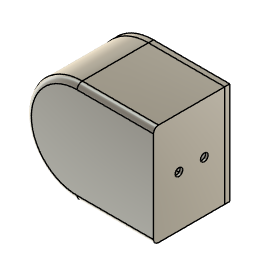
TRARM02_Link4 (Autodesk Fusion 360 design; units mm, degrees)
Autodesk Fusion 360 part; units mm, degrees
sketch "스케치1" plane through (0, 0, 0) normal (0, 0, 1) x (1, 0, 0) in component "TRARM02_Link4A_30x40x2 v1"
  line L0 (20, 30) -> (20, 0)
  line L1 (-20, 30) -> (-20, 0)
  arc A0 (-20, 0) -> (20, 0) centre (0, 0) ccw
  line L2 (-20, 30) -> (20, 30)
  dimension "d1" = 40
  dimension "d128" = 30
  dimension "d129" = 20
  constraint coincident A0.centre origin
  constraint tangent L0 A0
  constraint vertical L0
  constraint parallel L0 L1
  constraint horizontal L0.start L1.start
  measures "d1" diameter of A0
  measures "d128" vertical distance of A0.centre L1.start
  measures "d129" distance of A0.centre L1
extrude "돌출1" add sketch "스케치1" along normal blind 2 makes body 1 in component "TRARM02_Link4A_30x40x2 v1"
sketch "스케치2" plane through (0, 0, 2) normal (0, 0, 1) x (-1, 0, 0) in component "TRARM02_Link4A_30x40x2 v1"
  circle A0 centre (0, 8.75) radius 1.1
  circle A1 centre (0, -19.05) radius 1.1
  line L0 (6.1, -16.65) -> (-6.1, -16.65)
  line L1 (-6.1, -16.65) -> (-6.1, 6.35)
  line L2 (-6.1, 6.35) -> (6.1, 6.35)
  line L3 (6.1, 6.35) -> (6.1, -16.65)
  dimension "d7" = 2.2
  dimension "d8" = 27.8
  dimension "d9" = 8.75
  dimension "d11" = 23
  dimension "d12" = 2.4
  dimension "d13" = 12.2
  dimension "d14" = 6.1
  constraint equal A0 A1
  constraint horizontal L0
  constraint vertical L1
  constraint horizontal L2
  constraint vertical L3
  constraint vertical origin A0.centre
  constraint vertical origin A1.centre
  measures "d7" diameter of A0
  measures "d8" distance of A0.centre A1.centre
  measures "d9" distance of origin A0.centre
  measures "d11" distance of L0.end L1.end
  measures "d12" vertical distance of A1.centre L0.end
  measures "d13" distance of L0.start L0.end
  measures "d14" horizontal distance of origin L1.end
extrude "돌출2" cut sketch "스케치2" against normal blind 2 bodies 1 in component "TRARM02_Link4A_30x40x2 v1"
chamfer "챔퍼2" distance 1.5 angle 45 2 edges at (1.0256, 19.4478, 0) (1.0256, -8.3522, 0) on bodies 1 in component "TRARM02_Link4A_30x40x2 v1"
sketch "스케치14" plane through (0, 0, 2) normal (0, 0, 1) x (-1, 0, 0) in component "TRARM02_Link4A_30x40x2 v1"
  line L0 (20, -30) -> (20, 0) construction
  line L1 (-20, 0) -> (-20, -30) construction
  arc A0 (20, 0) -> (-20, 0) centre (0, 0) ccw construction
  line L2 (19, -29) -> (19, 0)
  arc A1 (19, 0) -> (-19, 0) centre (0, 0) ccw
  line L3 (-19, 0) -> (-19, -29)
  line L4 (-15, -6) -> (-18, -6)
  line L5 (15, -6) -> (18, -6)
  line L6 (15, 0) -> (18, 0)
  arc A2 (15, 0) -> (15, -6) centre (15, -3) ccw
  line L7 (18, -28) -> (18, -6)
  line L8 (-18, -6) -> (-18, -28)
  line L9 (-15, 0) -> (-18, 0)
  arc A3 (18, 0) -> (-18, 0) centre (0, 0) ccw
  arc A4 (-15, -6) -> (-15, 0) centre (-15, -3) ccw
  line L10 (-20, -30) -> (20, -30)
  line L11 (18, -28) -> (-18, -28)
  line L12 (19, -29) -> (-19, -29)
  dimension "d112" = 3
  dimension "d113" = 3
  dimension "d120" = 3
  dimension "d121" = 1
  dimension "d124" = 6
  dimension "d125" = 6
  dimension "d126" = 3
  dimension "d130" = 1
  dimension "d131" = 1
  constraint coincident L6.end L7
  constraint perpendicular L6 L7
  constraint coincident L6 A2.start
  constraint horizontal L5
  constraint vertical L6.start A2.centre
  constraint coincident L6.start A2.start
  constraint horizontal L4
  constraint horizontal L9
  constraint vertical L8
  constraint equal L4 L9
  constraint vertical L4.end L9.end
  constraint coincident A0.centre L6
  constraint coincident A0.centre L9
  constraint concentric A0 A3
  constraint concentric A0 A1
  constraint tangent L2 A1
  constraint tangent A1 L3
  constraint vertical L7
  constraint horizontal L12
  constraint horizontal L11
  measures "d112" distance of L5.start L5.end
  measures "d113" distance of L4.start L4.end
  measures "d120" distance of L6.start L6.end
  measures "d121" distance of L3 L8
  measures "d124" distance of A0.centre L5
  measures "d125" distance of A0.centre L4
  measures "d126" radius of A4
  measures "d130" distance of L11 L12
  measures "d131" distance of L10 L12
extrude "돌출15" add sketch "스케치14" along normal blind 2 bodies 1 in component "TRARM02_Link4A_30x40x2 v1"
sketch "스케치16" plane through (0, 0, 4) normal (0, 0, 1) x (-1, 0, 0) in component "TRARM02_Link4A_30x40x2 v1"
  circle A0 centre (-15, -3) radius 1.5
  circle A1 centre (15, -3) radius 1.5
  arc A2 (15, 0) -> (15, -6) centre (15, -3) ccw
  arc A3 (-15, -6) -> (-15, 0) centre (-15, -3) ccw
  dimension "d106" = 3
  constraint equal A0 A1
  constraint concentric A1 A2
  constraint concentric A0 A3
  measures "d106" diameter of A0
extrude "돌출17" cut sketch "스케치16" against normal blind 4 bodies 1 in component "TRARM02_Link4A_30x40x2 v1"
chamfer "챔퍼4" distance 2 angle 45 1 edges at (16.3985, 3.5424, 0) on bodies 1 in component "TRARM02_Link4A_30x40x2 v1"
chamfer "챔퍼4" distance 2 angle 45 1 edges at (-13.6015, 3.5424, 0) on bodies 1 in component "TRARM02_Link4A_30x40x2 v1"
move_body "이동1" bodies 1 to x (0, -1, 0) y (1, 0, 0) z (0, 0, 1) at (0, 0, 0) in component "TRARM02_Link4A_30x40x2 v1"
sketch "스케치1 (2)" plane through (0, 0, 0) normal (0, 0, 1) x (1, 0, 0) in component "TRARM02_Link4B_30x40x28 v1"
  line L0 (20, 30) -> (20, 0)
  line L1 (-20, 30) -> (-20, 0)
  arc A0 (-20, 0) -> (20, 0) centre (0, 0) ccw
  line L2 (-20, 30) -> (20, 30)
  dimension "d1_1" = 40
  dimension "d144" = 30
  constraint coincident A0.centre origin
  constraint tangent L0 A0
  constraint vertical L0
  constraint parallel L0 L1
  constraint horizontal L0.start L1.start
  measures "d1_1" diameter of A0
  measures "d144" vertical distance of A0.centre L1.start
extrude "돌출1'" add sketch "스케치1 (2)" along normal blind 2 separate body makes body 2 in component "TRARM02_Link4B_30x40x28 v1"
sketch "스케치14 (2)" plane through (0, 0, 2) normal (0, 0, 1) x (-1, 0, 0) in component "TRARM02_Link4B_30x40x28 v1"
  line L0 (20, -30) -> (20, 0)
  line L1 (-20, 0) -> (-20, -30)
  arc A0 (20, 0) -> (-20, 0) centre (0, 0) ccw
  arc A1 (19, 0) -> (-19, 0) centre (0, 0) ccw
  line L2 (15, -6) -> (19, -6)
  line L3 (15, 0) -> (19, 0)
  arc A2 (15, 0) -> (15, -6) centre (15, -3) ccw
  line L4 (-15, -6) -> (-19, -6)
  arc A3 (-15, -6) -> (-15, 0) centre (-15, -3) ccw
  line L5 (19, -29) -> (19, -6)
  line L6 (-19, -6) -> (-19, -29)
  line L7 (-15, 0) -> (-19, 0)
  line L8 (-20, -30) -> (20, -30)
  line L9 (20, -30) -> (-20, -30)
  line L10 (19, -29) -> (-19, -29)
  dimension "d111_1" = 15
  dimension "d112_1" = 6
  dimension "d114" = 3
  dimension "d132" = 4
  dimension "d133" = 4
  dimension "d134" = 4
  dimension "d135" = 1
  dimension "d136" = 4
  dimension "d142" = 1
  dimension "d143" = 19
  dimension "d145" = 1
  constraint concentric A0 A1
  constraint equal A2 A3
  constraint horizontal A2.centre A3.centre
  constraint horizontal L7
  constraint vertical L6
  constraint horizontal L4
  constraint vertical L5
  constraint horizontal L3
  constraint coincident A1.start L3.end
  constraint horizontal L2
  constraint coincident L0.start L8.end
  constraint coincident L1.end L8.start
  constraint horizontal L10
  measures "d111_1" horizontal distance of A0.centre A2.centre
  measures "d112_1" diameter of A2
  measures "d114" vertical distance of A0.centre A2.centre
  measures "d132" distance of L3.start A1.start
  measures "d133" distance of L2.start L2.end
  measures "d134" distance of A1.end A3.end
  measures "d135" distance of L1 L6
  measures "d136" distance of L4.start L4.end
  measures "d142" distance of L0 L5
  measures "d143" radius of A1
  measures "d145" distance of L9 L10
extrude "돌출18" add sketch "스케치14 (2)" along normal blind 26 bodies 2 in component "TRARM02_Link4B_30x40x28 v1"
sketch "스케치17" plane through (0, 0, 28) normal (0, 0, 1) x (-1, 0, 0) in component "TRARM02_Link4B_30x40x28 v1"
  line L0 (-19, -6) -> (-15, -6)
  line L1 (-15, 0) -> (-19, 0)
  arc A0 (-15, -6) -> (-15, 0) centre (-15, -3) ccw
  arc A1 (15, 0) -> (15, -6) centre (15, -3) ccw
  line L2 (19, 0) -> (15, 0)
  line L3 (15, -6) -> (19, -6)
  line L4 (19, -6) -> (19, 0)
  line L5 (-19, -6) -> (-19, 0)
  point P0 (15, 0)
  constraint coincident L3.end L4.start
  constraint coincident L2.start L4.end
  constraint coincident L0.start L5.start
  constraint coincident L1.end L5.end
extrude "돌출19" cut sketch "스케치17" against normal blind 2 bodies 2 in component "TRARM02_Link4B_30x40x28 v1"
sketch "스케치18" plane through (0, 0, 26) normal (0, 0, 1) x (-1, 0, 0) in component "TRARM02_Link4B_30x40x28 v1"
  circle A0 centre (15, -3) radius 1.45
  arc A1 (15, 0) -> (15, -6) centre (15, -3) ccw
  circle A2 centre (-15, -3) radius 1.45
  arc A3 (-15, -6) -> (-15, 0) centre (-15, -3) ccw
  constraint concentric A0 A1
  constraint equal A0 A2
extrude "돌출20" cut sketch "스케치18" against normal blind 5 bodies 2 in component "TRARM02_Link4B_30x40x28 v1"
fillet "필렛4" radius 2 3 edges at (20, 15, 0) (0, -20, 0) (-20, 15, 0) on bodies 2 in component "TRARM02_Link4B_30x40x28 v1"
sketch "스케치20" plane through (0, 0, 0) normal (0, 1, 0) x (1, 0, 0) in component "TRARM02_Link4B_30x40x28 v1"
  circle A0 centre (0, -15) radius 5
  dimension "d146" = 10
  dimension "d147" = 15
  constraint vertical origin A0.centre
  measures "d146" diameter of A0
  measures "d147" distance of origin A0.centre
extrude "돌출22" cut sketch "스케치20" against normal blind 40 bodies 2 in component "TRARM02_Link4B_30x40x28 v1"
sketch "스케치21" plane through (0, 30, 0) normal (0, 1, 0) x (-1, 0, 0) in component "TRARM02_Link4B_30x40x28 v1"
  circle A0 centre (0, 10) radius 1.5
  circle A1 centre (0, 20) radius 1.5
  dimension "d153" = 3
  dimension "d159" = 10
  dimension "d160" = 10
  constraint vertical origin A0.centre
  constraint equal A0 A1
  constraint vertical origin A1.centre
  measures "d153" diameter of A0
  measures "d159" distance of origin A0.centre
  measures "d160" distance of A0.centre A1.centre
extrude "돌출23" cut sketch "스케치21" against normal blind 1 bodies 2 in component "TRARM02_Link4B_30x40x28 v1"
move_body "이동1'" bodies 2 to x (0, 0, -1) y (0, 1, 0) z (1, 0, 0) at (-30, 0, 30) in component "TRARM02_Link4B_30x40x28 v1"
move_body "이동2" bodies 1 to x (1, 0, 0) y (0, 0, 1) z (0, -1, 0) at (0, 0, 0) in component "TRARM02_Link4A_30x40x2 v1"
component "TRARM02_Link4A_30x40x2 v1" placed x (1, 0, 0) y (0, 1, 0) z (0, 0, 1) at (0, 0, 0)
component "TRARM02_Link4B_30x40x28 v1" placed x (0, 1, 0) y (1, 0, 0) z (0, 0, -1) at (0, 0, 30)
